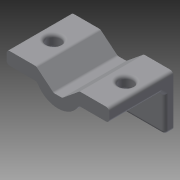
# Autodesk Inventor part: rodClamp
Saved by Autodesk Inventor 2014 (Build 180170000, 170)
## iProperties
Created: 2014-01-10
Part Number: rodClamp
Material: Generic
Document SubType Name: Modeling
Designer: Peele
Density: 1 g/cm^3
Appearance: Default
Author: Peele
Autodesk Inventor part; units mm, degrees
ref_plane "YZ Plane" through (0, 0, 0) normal (1, 0, 0) x (0, 1, 0)
ref_plane "XZ Plane" through (0, 0, 0) normal (0, 1, 0) x (-1, 0, 0)
ref_plane "XY Plane" through (0, 0, 0) normal (0, 0, 1) x (1, 0, 0)
sketch "Sketch1" plane through (0, 0, 0) normal (0, 0, 1) x (1, 0, 0)
  line L0 (-10, -12.5) -> (10, -12.5) construction
  line L1 (10, -12.5) -> (10, 12.5) construction
  line L2 (10, 12.5) -> (-10, 12.5) construction
  line L3 (-10, 12.5) -> (-10, -12.5) construction
  line L4 (-10, -12.5) -> (10, 12.5) construction
  line L5 (10, -12.5) -> (-10, 12.5) construction
  circle A0 centre (-10, 12.5) radius 1.925
  circle A1 centre (10, 12.5) radius 1.925
  circle A2 centre (10, -12.5) radius 1.925
  circle A3 centre (-10, -12.5) radius 1.925
  arc A4 (-7.1685, 17.7046) -> (-15.1908, 9.6432) centre (-10, 12.5) ccw
  arc A5 (15.1908, 9.6432) -> (7.1685, 17.7046) centre (10, 12.5) ccw
  arc A6 (7.1685, -17.7046) -> (15.1908, -9.6432) centre (10, -12.5) ccw
  arc A7 (-15.1908, -9.6432) -> (-7.1685, -17.7046) centre (-10, -12.5) ccw
  arc A8 (-7.1685, 17.7046) -> (7.1685, 17.7046) centre (0, 30.8808) ccw
  arc A9 (7.1685, -17.7046) -> (-7.1685, -17.7046) centre (0, -30.8808) ccw
  arc A10 (15.1908, 9.6432) -> (15.1908, -9.6432) centre (32.7125, 0) ccw
  arc A11 (-15.1908, -9.6432) -> (-15.1908, 9.6432) centre (-32.7125, 0) ccw
  point P0 (0, 0)
  dimension "d0" = 25
  dimension "d1" = 20
  dimension "d2" = 3.85
  dimension "d3" = 4
  dimension "d4" = 15
  dimension "d5" = 20
  constraints: 16 point on circle, 12 centre point, 12 end point, 8 coincident, 8 equal radius, 8 tangent, 2 midpoint, 2 parallel, 1 horizontal, 1 perpendicular
  measures "d0" distance of L2.end L0.start
  measures "d1" distance of L1.end L2.end
  measures "d2" diameter of A0
  measures "d3" radial gap between concentric circles of A4 A0
  measures "d4" radius of A8
  measures "d5" radius of A11
extrude "Extrusion1" add sketch "Sketch1" along normal blind 5
sketch "Sketch2" plane through (0, 0, 5) normal (0, 0, 1) x (1, 0, 0)
  circle A0 centre (0, 0) radius 4 construction
  line L0 (-1, -4.35) -> (1, -4.35)
  line L1 (1, -4.35) -> (5.0946, -1)
  line L2 (5.0946, -1) -> (12, -1)
  line L3 (-1, -4.35) -> (-5.0946, -1)
  line L4 (-5.0946, -1) -> (-12, -1)
  line L5 (0, 0) -> (0, -4.35) construction
  line L6 (-12, -1) -> (-12, -4)
  line L7 (-12, -4) -> (-4.899, -4)
  line L8 (12, -1) -> (12, -4)
  line L9 (12, -4) -> (4.899, -4)
  arc A1 (-4.899, -4) -> (4.899, -4) centre (0, -1.5) ccw
  dimension "d8" = 8
  dimension "d9" = 1
  dimension "d10" = 3
  dimension "d11" = 24
  dimension "d12" = 2
  dimension "d13" = 3.35
  dimension "d14" = 5.5
  dimension "d15" = 2.5
  constraints: 20 end point, 3 equal length, 3 perpendicular, 2 centre point, 2 collinear, 2 parallel, 2 point on circle, 2 tangent, 1 coincident, 1 horizontal, 1 midpoint, 1 vertical
  measures "d8" diameter of A0
  measures "d9" distance from line of point (0, 0) L4
  measures "d10" distance of L4.end L6.end
  measures "d11" distance between parallel lines of L8 L6
  measures "d12" distance of L0.start L0.end
  measures "d13" distance between parallel lines of L2 L0
  measures "d14" radius of A1
  measures "d15" distance from line of A1.centre L9
extrude "Extrusion2" add sketch "Sketch2" along normal blind 15
sketch "Sketch3" plane through (4.899, -4, 5) normal (0, -1, 0) x (1, 0, 0)
  line L0 (7.101, 0) -> (0, 0) projected
  line L1 (7.101, 0) -> (7.101, 15) projected
  line L2 (0, 0) -> (0, 15) projected
  circle A0 centre (3.5505, 7.5) radius 1.6
  circle A1 centre (-13.3485, 7.5) radius 1.6
  line L3 (3.5505, 0) -> (3.5505, 7.5) construction
  line L4 (3.5505, 7.5) -> (7.101, 7.5) construction
  line L5 (-16.899, 7.5) -> (-13.3485, 7.5) construction
  line L6 (-13.3485, 7.5) -> (-13.3485, 0) construction
  line L7 (-16.899, 0) -> (-16.899, 15) projected
  point P0 (-4.899, -5)
  dimension "d18" = 3.2
  constraints: 8 end point, 3 midpoint, 2 centre point, 2 collinear, 2 equal length, 1 coincident, 1 equal radius, 1 horizontal, 1 parallel, 1 perpendicular
  measures "d18" diameter of A0
extrude "Extrusion3" cut sketch "Sketch3" against normal blind 15
sketch "Sketch4" plane through (0, 0, 5) normal (0, 0, 1) x (1, 0, 0)
  line L0 (1, -4.35) -> (5.0946, -1) projected
  line L1 (-5.0946, -1) -> (-1, -4.35) projected
  line L2 (-1, -4.35) -> (1, -4.35) projected
  line L3 (-5.0946, -1) -> (-1, -4.35)
  line L4 (-1, -4.35) -> (1, -4.35)
  line L5 (1, -4.35) -> (5.0946, -1)
  line L6 (5.0946, 21.1209) -> (-5.0946, 21.1209)
  line L7 (-5.0946, 21.1209) -> (-5.0946, -1)
  line L8 (5.0946, -1) -> (5.0946, 21.1209)
  point P0 (0, 0)
  constraints: 12 end point, 3 collinear, 2 parallel, 1 perpendicular
extrude "Extrusion4" cut sketch "Sketch4" against normal blind 10
sketch "Sketch5" plane through (-12, -1, 20) normal (0, 1, 0) x (1, 0, 0)
  line L0 (0, 15) -> (6.9054, 15) projected
  line L1 (-11.2791, 15) -> (33.3469, 15)
  line L2 (33.3469, 15) -> (33.3469, 24.5778)
  line L3 (33.3469, 24.5778) -> (-11.2791, 24.5778)
  line L4 (-11.2791, 24.5778) -> (-11.2791, 15)
  point P0 (12, 20)
  constraints: 8 end point, 2 parallel, 1 collinear, 1 horizontal, 1 perpendicular
extrude "Extrusion5" cut sketch "Sketch5" against normal blind 25.875 and the other way blind 28.8125
sketch "Sketch6" plane through (-5.0946, -1, 5) normal (0, 0, -1) x (-1, 0, 0)
  line L0 (-10.1893, 0) -> (-6.0946, -3.35) projected
  line L1 (-10.1893, 0) -> (-17.0946, 0) projected
  line L2 (-17.0946, 0) -> (-17.0946, -3) projected
  line L3 (-17.0946, -3) -> (-9.9936, -3) projected
  arc A0 (-9.9936, -3) -> (-0.1957, -3) centre (-5.0946, -0.5) ccw projected
  line L4 (-0.1957, -3) -> (6.9054, -3) projected
  line L5 (6.9054, -3) -> (6.9054, 0) projected
  line L6 (6.9054, 0) -> (0, 0) projected
  line L7 (-4.0946, -3.35) -> (0, 0) projected
  line L8 (-6.0946, -3.35) -> (-4.0946, -3.35) projected
  line L9 (-17.0946, 0) -> (-10.1893, 0)
  line L10 (-6.0946, -3.35) -> (-10.1893, 0)
  line L11 (-6.0946, -3.35) -> (-4.0946, -3.35)
  line L12 (-4.0946, -3.35) -> (0, 0)
  line L13 (0, 0) -> (6.9054, 0)
  line L14 (6.9054, 0) -> (6.9054, -12)
  line L15 (6.9054, -12) -> (-17.0946, -12)
  line L16 (-17.0946, -12) -> (-17.0946, 0)
  point P0 (-5.0946, 1)
  dimension "d36" = 12
  constraints: 16 end point, 4 collinear, 2 parallel, 1 perpendicular, 1 point on line
  measures "d36" distance of L5.end L14.end
extrude "Extrusion6" add sketch "Sketch6" against normal blind 2 contours L3 A0 L4 L14 L15 L16
chamfer "Chamfer2" distance 1 angle 45 3 edges at (-8.4495, -4, 7) (0, -7, 7) (8.4495, -4, 7)
fillet "Fillet6" radius 0.75 21 edges at (12, -4, 14) (12, -1, 12.5) (-12, -4, 14) (-12, -1, 12.5) (-4.899, -4, 14) (4.899, -4, 14) (5.0946, -1, 12.5) (1, -4.35, 12.5) (-1, -4.35, 12.5) (-5.0946, -1, 12.5) (6.8495, -4, 12.5) (6.8495, -1, 12.5) (-10.0495, -4, 12.5) (-10.0495, -1, 12.5) (-12, -4.5, 7.5) (-12, -9, 7) (12, -4.5, 7.5) (12, -9, 7) (0, -13, 7) (12, -13, 6) (-12, -13, 6)
body "Solid1"
